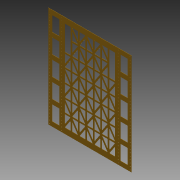
# Autodesk Inventor part: Cover Nick
Saved by Autodesk Inventor 2014 SP1 (Build 180222100, 222)
## iProperties
Created: 2014-01-21
Part Number: Cover Nick
Material: Aluminum 6061
Document SubType Name: Sheet Metal
Designer: Nick
Density: 2.71 g/cm^3
Sheet Metal Rule: Default
Appearance: Brass - Satin
Mass: 2078.93 g
Surface Area: 7373.94 cm^2
Volume: 767.135 cm^3
Author: Nick
Autodesk Inventor part; units mm, degrees
(part 1 of 2)
ref_plane "YZ Plane" through (0, 0, 0) normal (1, 0, 0) x (0, 1, 0)
ref_plane "XZ Plane" through (0, 0, 0) normal (0, 1, 0) x (-1, 0, 0)
ref_plane "XY Plane" through (0, 0, 0) normal (0, 0, 1) x (1, 0, 0)
sketch "Sketch1" plane through (0, 0, 0) normal (0, 0, 1) x (1, 0, 0)
  line L0 (0, 0) -> (711.2, 0)
  line L1 (711.2, 0) -> (711.2, -863.6)
  line L2 (711.2, -863.6) -> (0, -863.6)
  line L3 (0, -863.6) -> (0, 0)
  line L4 (139.7, -50.0761) -> (139.7, -112.6148)
  line L5 (145.5168, -114.376) -> (187.2092, -51.8373)
  line L6 (184.5675, -46.9011) -> (142.875, -46.9011)
  line L7 (190.5, -69.7865) -> (190.5, -142.8115)
  line L8 (187.325, -145.9865) -> (145.6325, -145.9865)
  line L9 (142.9908, -141.0503) -> (190.5, -69.7865)
  line L10 (196.85, 58.9554) -> (196.85, -325.5512) construction
  line L11 (254, -50.0761) -> (254, -112.6148)
  line L12 (248.1832, -114.376) -> (206.4908, -51.8373)
  line L13 (209.1325, -46.9011) -> (250.825, -46.9011)
  line L14 (203.2, -80.2728) -> (203.2, -142.8115)
  line L15 (206.375, -145.9865) -> (248.0675, -145.9865)
  line L16 (250.7092, -141.0503) -> (209.0168, -78.5116)
  arc A0 (142.875, -46.9011) -> (139.7, -50.0761) centre (142.875, -50.0761) ccw
  arc A1 (139.7, -112.6148) -> (145.5168, -114.376) centre (142.875, -112.6148) ccw
  arc A2 (187.2092, -51.8373) -> (184.5675, -46.9011) centre (184.5675, -50.0761) ccw
  arc A3 (209.1325, -46.9011) -> (206.4908, -51.8373) centre (209.1325, -50.0761) ccw
  arc A4 (254, -50.0761) -> (250.825, -46.9011) centre (250.825, -50.0761) ccw
  arc A5 (248.1832, -114.376) -> (254, -112.6148) centre (250.825, -112.6148) ccw
  arc A6 (248.0675, -145.9865) -> (250.7092, -141.0503) centre (248.0675, -142.8115) ccw
  arc A7 (209.0168, -78.5116) -> (203.2, -80.2728) centre (206.375, -80.2728) ccw
  arc A8 (203.2, -142.8115) -> (206.375, -145.9865) centre (206.375, -142.8115) ccw
  arc A9 (187.325, -145.9865) -> (190.5, -142.8115) centre (187.325, -142.8115) ccw
  arc A10 (142.9908, -141.0503) -> (145.6325, -145.9865) centre (145.6325, -142.8115) ccw
  line L17 (88.986, -152.3365) -> (322.9088, -152.3365) construction
  line L18 (139.7, -254.5969) -> (139.7, -192.0582)
  line L19 (145.5168, -190.297) -> (187.2092, -252.8357)
  line L20 (184.5675, -257.7719) -> (142.875, -257.7719)
  line L21 (190.5, -234.8865) -> (190.5, -161.8615)
  line L22 (187.325, -158.6865) -> (145.6325, -158.6865)
  line L23 (142.9908, -163.6227) -> (190.5, -234.8865)
  line L24 (209.1325, -257.7719) -> (250.825, -257.7719)
  line L25 (254, -254.5969) -> (254, -192.0582)
  line L26 (248.1832, -190.297) -> (206.4908, -252.8357)
  line L27 (206.375, -158.6865) -> (248.0675, -158.6865)
  line L28 (250.7092, -163.6227) -> (209.0168, -226.1614)
  line L29 (203.2, -224.4002) -> (203.2, -161.8615)
  arc A11 (139.7, -254.5969) -> (142.875, -257.7719) centre (142.875, -254.5969) ccw
  arc A12 (145.5168, -190.297) -> (139.7, -192.0582) centre (142.875, -192.0582) ccw
  arc A13 (184.5675, -257.7719) -> (187.2092, -252.8357) centre (184.5675, -254.5969) ccw
  arc A14 (206.4908, -252.8357) -> (209.1325, -257.7719) centre (209.1325, -254.5969) ccw
  arc A15 (250.825, -257.7719) -> (254, -254.5969) centre (250.825, -254.5969) ccw
  arc A16 (254, -192.0582) -> (248.1832, -190.297) centre (250.825, -192.0582) ccw
  arc A17 (250.7092, -163.6227) -> (248.0675, -158.6865) centre (248.0675, -161.8615) ccw
  arc A18 (203.2, -224.4002) -> (209.0168, -226.1614) centre (206.375, -224.4002) ccw
  arc A19 (206.375, -158.6865) -> (203.2, -161.8615) centre (206.375, -161.8615) ccw
  arc A20 (190.5, -161.8615) -> (187.325, -158.6865) centre (187.325, -161.8615) ccw
  arc A21 (145.6325, -158.6865) -> (142.9908, -163.6227) centre (145.6325, -161.8615) ccw
  line L30 (266.7, -50.0761) -> (266.7, -112.6148)
  line L31 (272.5168, -114.376) -> (314.2092, -51.8373)
  line L32 (311.5675, -46.9011) -> (269.875, -46.9011)
  line L33 (317.5, -69.7865) -> (317.5, -142.8115)
  line L34 (314.325, -145.9865) -> (272.6325, -145.9865)
  line L35 (269.9908, -141.0503) -> (317.5, -69.7865)
  line L36 (336.1325, -46.9011) -> (377.825, -46.9011)
  line L37 (381, -50.0761) -> (381, -112.6148)
  line L38 (375.1832, -114.376) -> (333.4908, -51.8373)
  line L39 (333.375, -145.9865) -> (375.0675, -145.9865)
  line L40 (377.7092, -141.0503) -> (336.0168, -78.5116)
  line L41 (330.2, -80.2728) -> (330.2, -142.8115)
  arc A22 (269.875, -46.9011) -> (266.7, -50.0761) centre (269.875, -50.0761) ccw
  arc A23 (266.7, -112.6148) -> (272.5168, -114.376) centre (269.875, -112.6148) ccw
  arc A24 (314.2092, -51.8373) -> (311.5675, -46.9011) centre (311.5675, -50.0761) ccw
  arc A25 (336.1325, -46.9011) -> (333.4908, -51.8373) centre (336.1325, -50.0761) ccw
  arc A26 (381, -50.0761) -> (377.825, -46.9011) centre (377.825, -50.0761) ccw
  arc A27 (375.1832, -114.376) -> (381, -112.6148) centre (377.825, -112.6148) ccw
  arc A28 (375.0675, -145.9865) -> (377.7092, -141.0503) centre (375.0675, -142.8115) ccw
  arc A29 (336.0168, -78.5116) -> (330.2, -80.2728) centre (333.375, -80.2728) ccw
  arc A30 (330.2, -142.8115) -> (333.375, -145.9865) centre (333.375, -142.8115) ccw
  arc A31 (314.325, -145.9865) -> (317.5, -142.8115) centre (314.325, -142.8115) ccw
  arc A32 (269.9908, -141.0503) -> (272.6325, -145.9865) centre (272.6325, -142.8115) ccw
  line L42 (317.5, -234.8865) -> (317.5, -161.8615)
  line L43 (269.9908, -163.6227) -> (317.5, -234.8865)
  line L44 (272.5168, -190.297) -> (314.2092, -252.8357)
  line L45 (311.5675, -257.7719) -> (269.875, -257.7719)
  line L46 (266.7, -254.5969) -> (266.7, -192.0582)
  line L47 (330.2, -224.4002) -> (330.2, -161.8615)
  line L48 (314.325, -158.6865) -> (272.6325, -158.6865)
  arc A33 (317.5, -161.8615) -> (314.325, -158.6865) centre (314.325, -161.8615) ccw
  arc A34 (272.5168, -190.297) -> (266.7, -192.0582) centre (269.875, -192.0582) ccw
  arc A35 (272.6325, -158.6865) -> (269.9908, -163.6227) centre (272.6325, -161.8615) ccw
  arc A36 (330.2, -224.4002) -> (336.0168, -226.1614) centre (333.375, -224.4002) ccw
  arc A37 (333.375, -158.6865) -> (330.2, -161.8615) centre (333.375, -161.8615) ccw
  line L49 (375.1832, -190.297) -> (333.4908, -252.8357)
  line L50 (381, -254.5969) -> (381, -192.0582)
  line L51 (377.7092, -163.6227) -> (336.0168, -226.1614)
  line L52 (333.375, -158.6865) -> (375.0675, -158.6865)
  arc A38 (381, -192.0582) -> (375.1832, -190.297) centre (377.825, -192.0582) ccw
  arc A39 (377.7092, -163.6227) -> (375.0675, -158.6865) centre (375.0675, -161.8615) ccw
  arc A40 (266.7, -254.5969) -> (269.875, -257.7719) centre (269.875, -254.5969) ccw
  line L53 (336.1325, -257.7719) -> (377.825, -257.7719)
  arc A41 (311.5675, -257.7719) -> (314.2092, -252.8357) centre (311.5675, -254.5969) ccw
  arc A42 (377.825, -257.7719) -> (381, -254.5969) centre (377.825, -254.5969) ccw
  arc A43 (333.4908, -252.8357) -> (336.1325, -257.7719) centre (336.1325, -254.5969) ccw
  line L54 (393.7, -50.0761) -> (393.7, -112.6148)
  line L55 (399.5168, -114.376) -> (441.2092, -51.8373)
  line L56 (438.5675, -46.9011) -> (396.875, -46.9011)
  line L57 (444.5, -69.7865) -> (444.5, -142.8115)
  line L58 (441.325, -145.9865) -> (399.6325, -145.9865)
  line L59 (396.9908, -141.0503) -> (444.5, -69.7865)
  line L60 (463.1325, -46.9011) -> (504.825, -46.9011)
  line L61 (508, -50.0761) -> (508, -112.6148)
  line L62 (502.1832, -114.376) -> (460.4908, -51.8373)
  line L63 (460.375, -145.9865) -> (502.0675, -145.9865)
  line L64 (504.7092, -141.0503) -> (463.0168, -78.5116)
  line L65 (457.2, -80.2728) -> (457.2, -142.8115)
  arc A44 (396.875, -46.9011) -> (393.7, -50.0761) centre (396.875, -50.0761) ccw
  arc A45 (393.7, -112.6148) -> (399.5168, -114.376) centre (396.875, -112.6148) ccw
  arc A46 (441.2092, -51.8373) -> (438.5675, -46.9011) centre (438.5675, -50.0761) ccw
  arc A47 (463.1325, -46.9011) -> (460.4908, -51.8373) centre (463.1325, -50.0761) ccw
  arc A48 (508, -50.0761) -> (504.825, -46.9011) centre (504.825, -50.0761) ccw
  arc A49 (502.1832, -114.376) -> (508, -112.6148) centre (504.825, -112.6148) ccw
  arc A50 (502.0675, -145.9865) -> (504.7092, -141.0503) centre (502.0675, -142.8115) ccw
  arc A51 (463.0168, -78.5116) -> (457.2, -80.2728) centre (460.375, -80.2728) ccw
  arc A52 (457.2, -142.8115) -> (460.375, -145.9865) centre (460.375, -142.8115) ccw
  arc A53 (441.325, -145.9865) -> (444.5, -142.8115) centre (441.325, -142.8115) ccw
  arc A54 (396.9908, -141.0503) -> (399.6325, -145.9865) centre (399.6325, -142.8115) ccw
  line L66 (444.5, -234.8865) -> (444.5, -161.8615)
  line L67 (396.9908, -163.6227) -> (444.5, -234.8865)
  line L68 (399.5168, -190.297) -> (441.2092, -252.8357)
  line L69 (438.5675, -257.7719) -> (396.875, -257.7719)
  line L70 (393.7, -254.5969) -> (393.7, -192.0582)
  line L71 (457.2, -224.4002) -> (457.2, -161.8615)
  line L72 (441.325, -158.6865) -> (399.6325, -158.6865)
  arc A55 (444.5, -161.8615) -> (441.325, -158.6865) centre (441.325, -161.8615) ccw
  arc A56 (399.5168, -190.297) -> (393.7, -192.0582) centre (396.875, -192.0582) ccw
  arc A57 (399.6325, -158.6865) -> (396.9908, -163.6227) centre (399.6325, -161.8615) ccw
  arc A58 (457.2, -224.4002) -> (463.0168, -226.1614) centre (460.375, -224.4002) ccw
  arc A59 (460.375, -158.6865) -> (457.2, -161.8615) centre (460.375, -161.8615) ccw
  line L73 (502.1832, -190.297) -> (460.4908, -252.8357)
  line L74 (508, -254.5969) -> (508, -192.0582)
  line L75 (504.7092, -163.6227) -> (463.0168, -226.1614)
  line L76 (460.375, -158.6865) -> (502.0675, -158.6865)
  arc A60 (508, -192.0582) -> (502.1832, -190.297) centre (504.825, -192.0582) ccw
  arc A61 (504.7092, -163.6227) -> (502.0675, -158.6865) centre (502.0675, -161.8615) ccw
  arc A62 (393.7, -254.5969) -> (396.875, -257.7719) centre (396.875, -254.5969) ccw
  line L77 (463.1325, -257.7719) -> (504.825, -257.7719)
  arc A63 (438.5675, -257.7719) -> (441.2092, -252.8357) centre (438.5675, -254.5969) ccw
  arc A64 (504.825, -257.7719) -> (508, -254.5969) centre (504.825, -254.5969) ccw
  arc A65 (460.4908, -252.8357) -> (463.1325, -257.7719) centre (463.1325, -254.5969) ccw
  line L78 (139.7, -273.6469) -> (139.7, -336.1856)
  line L79 (145.5168, -337.9468) -> (187.2092, -275.4081)
  line L80 (184.5675, -270.4719) -> (142.875, -270.4719)
  line L81 (190.5, -293.3573) -> (190.5, -366.3823)
  line L82 (187.325, -369.5573) -> (145.6325, -369.5573)
  line L83 (142.9908, -364.6211) -> (190.5, -293.3573)
  line L84 (209.1325, -270.4719) -> (250.825, -270.4719)
  line L85 (254, -273.6469) -> (254, -336.1856)
  line L86 (248.1832, -337.9468) -> (206.4908, -275.4081)
  line L87 (206.375, -369.5573) -> (248.0675, -369.5573)
  line L88 (250.7092, -364.6211) -> (209.0168, -302.0824)
  line L89 (203.2, -303.8436) -> (203.2, -366.3823)
  arc A66 (142.875, -270.4719) -> (139.7, -273.6469) centre (142.875, -273.6469) ccw
  arc A67 (139.7, -336.1856) -> (145.5168, -337.9468) centre (142.875, -336.1856) ccw
  arc A68 (187.2092, -275.4081) -> (184.5675, -270.4719) centre (184.5675, -273.6469) ccw
  arc A69 (209.1325, -270.4719) -> (206.4908, -275.4081) centre (209.1325, -273.6469) ccw
  arc A70 (254, -273.6469) -> (250.825, -270.4719) centre (250.825, -273.6469) ccw
  arc A71 (248.1832, -337.9468) -> (254, -336.1856) centre (250.825, -336.1856) ccw
  arc A72 (248.0675, -369.5573) -> (250.7092, -364.6211) centre (248.0675, -366.3823) ccw
  arc A73 (209.0168, -302.0824) -> (203.2, -303.8436) centre (206.375, -303.8436) ccw
  arc A74 (203.2, -366.3823) -> (206.375, -369.5573) centre (206.375, -366.3823) ccw
  arc A75 (187.325, -369.5573) -> (190.5, -366.3823) centre (187.325, -366.3823) ccw
  arc A76 (142.9908, -364.6211) -> (145.6325, -369.5573) centre (145.6325, -366.3823) ccw
  line L90 (190.5, -458.4573) -> (190.5, -385.4323)
  line L91 (142.9908, -387.1935) -> (190.5, -458.4573)
  line L92 (145.5168, -413.8678) -> (187.2092, -476.4065)
  line L93 (184.5675, -481.3427) -> (142.875, -481.3427)
  line L94 (139.7, -478.1677) -> (139.7, -415.629)
  line L95 (203.2, -447.971) -> (203.2, -385.4323)
  line L96 (187.325, -382.2573) -> (145.6325, -382.2573)
  arc A77 (190.5, -385.4323) -> (187.325, -382.2573) centre (187.325, -385.4323) ccw
  arc A78 (145.5168, -413.8678) -> (139.7, -415.629) centre (142.875, -415.629) ccw
  arc A79 (145.6325, -382.2573) -> (142.9908, -387.1935) centre (145.6325, -385.4323) ccw
  arc A80 (203.2, -447.971) -> (209.0168, -449.7322) centre (206.375, -447.971) ccw
  arc A81 (206.375, -382.2573) -> (203.2, -385.4323) centre (206.375, -385.4323) ccw
  line L97 (248.1832, -413.8678) -> (206.4908, -476.4065)
  line L98 (254, -478.1677) -> (254, -415.629)
  line L99 (250.7092, -387.1935) -> (209.0168, -449.7322)
  line L100 (206.375, -382.2573) -> (248.0675, -382.2573)
  arc A82 (254, -415.629) -> (248.1832, -413.8678) centre (250.825, -415.629) ccw
  arc A83 (250.7092, -387.1935) -> (248.0675, -382.2573) centre (248.0675, -385.4323) ccw
  arc A84 (139.7, -478.1677) -> (142.875, -481.3427) centre (142.875, -478.1677) ccw
  line L101 (209.1325, -481.3427) -> (250.825, -481.3427)
  arc A85 (184.5675, -481.3427) -> (187.2092, -476.4065) centre (184.5675, -478.1677) ccw
  arc A86 (250.825, -481.3427) -> (254, -478.1677) centre (250.825, -478.1677) ccw
  arc A87 (206.4908, -476.4065) -> (209.1325, -481.3427) centre (209.1325, -478.1677) ccw
  line L102 (266.7, -273.6469) -> (266.7, -336.1856)
  line L103 (272.5168, -337.9468) -> (314.2092, -275.4081)
  line L104 (311.5675, -270.4719) -> (269.875, -270.4719)
  line L105 (317.5, -293.3573) -> (317.5, -366.3823)
  line L106 (314.325, -369.5573) -> (272.6325, -369.5573)
  line L107 (269.9908, -364.6211) -> (317.5, -293.3573)
  line L108 (336.1325, -270.4719) -> (377.825, -270.4719)
  line L109 (381, -273.6469) -> (381, -336.1856)
  line L110 (375.1832, -337.9468) -> (333.4908, -275.4081)
  line L111 (333.375, -369.5573) -> (375.0675, -369.5573)
  line L112 (377.7092, -364.6211) -> (336.0168, -302.0824)
  line L113 (330.2, -303.8436) -> (330.2, -366.3823)
  arc A88 (269.875, -270.4719) -> (266.7, -273.6469) centre (269.875, -273.6469) ccw
  arc A89 (266.7, -336.1856) -> (272.5168, -337.9468) centre (269.875, -336.1856) ccw
  arc A90 (314.2092, -275.4081) -> (311.5675, -270.4719) centre (311.5675, -273.6469) ccw
  arc A91 (336.1325, -270.4719) -> (333.4908, -275.4081) centre (336.1325, -273.6469) ccw
  arc A92 (381, -273.6469) -> (377.825, -270.4719) centre (377.825, -273.6469) ccw
  arc A93 (375.1832, -337.9468) -> (381, -336.1856) centre (377.825, -336.1856) ccw
  arc A94 (375.0675, -369.5573) -> (377.7092, -364.6211) centre (375.0675, -366.3823) ccw
  arc A95 (336.0168, -302.0824) -> (330.2, -303.8436) centre (333.375, -303.8436) ccw
  arc A96 (330.2, -366.3823) -> (333.375, -369.5573) centre (333.375, -366.3823) ccw
  arc A97 (314.325, -369.5573) -> (317.5, -366.3823) centre (314.325, -366.3823) ccw
  arc A98 (269.9908, -364.6211) -> (272.6325, -369.5573) centre (272.6325, -366.3823) ccw
  line L114 (317.5, -458.4573) -> (317.5, -385.4323)
  line L115 (269.9908, -387.1935) -> (317.5, -458.4573)
  line L116 (272.5168, -413.8678) -> (314.2092, -476.4065)
  line L117 (311.5675, -481.3427) -> (269.875, -481.3427)
  line L118 (266.7, -478.1677) -> (266.7, -415.629)
  line L119 (330.2, -447.971) -> (330.2, -385.4323)
  line L120 (314.325, -382.2573) -> (272.6325, -382.2573)
  arc A99 (317.5, -385.4323) -> (314.325, -382.2573) centre (314.325, -385.4323) ccw
  arc A100 (272.5168, -413.8678) -> (266.7, -415.629) centre (269.875, -415.629) ccw
  arc A101 (272.6325, -382.2573) -> (269.9908, -387.1935) centre (272.6325, -385.4323) ccw
  arc A102 (330.2, -447.971) -> (336.0168, -449.7322) centre (333.375, -447.971) ccw
  arc A103 (333.375, -382.2573) -> (330.2, -385.4323) centre (333.375, -385.4323) ccw
  line L121 (375.1832, -413.8678) -> (333.4908, -476.4065)
  line L122 (381, -478.1677) -> (381, -415.629)
  line L123 (377.7092, -387.1935) -> (336.0168, -449.7322)
  line L124 (333.375, -382.2573) -> (375.0675, -382.2573)
  arc A104 (381, -415.629) -> (375.1832, -413.8678) centre (377.825, -415.629) ccw
  arc A105 (377.7092, -387.1935) -> (375.0675, -382.2573) centre (375.0675, -385.4323) ccw
  arc A106 (266.7, -478.1677) -> (269.875, -481.3427) centre (269.875, -478.1677) ccw
  line L125 (336.1325, -481.3427) -> (377.825, -481.3427)
  arc A107 (311.5675, -481.3427) -> (314.2092, -476.4065) centre (311.5675, -478.1677) ccw
  arc A108 (377.825, -481.3427) -> (381, -478.1677) centre (377.825, -478.1677) ccw
  arc A109 (333.4908, -476.4065) -> (336.1325, -481.3427) centre (336.1325, -478.1677) ccw
  line L126 (393.7, -273.6469) -> (393.7, -336.1856)
  line L127 (399.5168, -337.9468) -> (441.2092, -275.4081)
  line L128 (438.5675, -270.4719) -> (396.875, -270.4719)
  line L129 (444.5, -293.3573) -> (444.5, -366.3823)
  line L130 (441.325, -369.5573) -> (399.6325, -369.5573)
  line L131 (396.9908, -364.6211) -> (444.5, -293.3573)
  line L132 (463.1325, -270.4719) -> (504.825, -270.4719)
  line L133 (508, -273.6469) -> (508, -336.1856)
  line L134 (502.1832, -337.9468) -> (460.4908, -275.4081)
  line L135 (460.375, -369.5573) -> (502.0675, -369.5573)
  line L136 (504.7092, -364.6211) -> (463.0168, -302.0824)
  line L137 (457.2, -303.8436) -> (457.2, -366.3823)
  arc A110 (396.875, -270.4719) -> (393.7, -273.6469) centre (396.875, -273.6469) ccw
  arc A111 (393.7, -336.1856) -> (399.5168, -337.9468) centre (396.875, -336.1856) ccw
  arc A112 (441.2092, -275.4081) -> (438.5675, -270.4719) centre (438.5675, -273.6469) ccw
  arc A113 (463.1325, -270.4719) -> (460.4908, -275.4081) centre (463.1325, -273.6469) ccw
  arc A114 (508, -273.6469) -> (504.825, -270.4719) centre (504.825, -273.6469) ccw
  arc A115 (502.1832, -337.9468) -> (508, -336.1856) centre (504.825, -336.1856) ccw
  arc A116 (502.0675, -369.5573) -> (504.7092, -364.6211) centre (502.0675, -366.3823) ccw
  arc A117 (463.0168, -302.0824) -> (457.2, -303.8436) centre (460.375, -303.8436) ccw
  arc A118 (457.2, -366.3823) -> (460.375, -369.5573) centre (460.375, -366.3823) ccw
  arc A119 (441.325, -369.5573) -> (444.5, -366.3823) centre (441.325, -366.3823) ccw
  arc A120 (396.9908, -364.6211) -> (399.6325, -369.5573) centre (399.6325, -366.3823) ccw
  line L138 (444.5, -458.4573) -> (444.5, -385.4323)
  line L139 (396.9908, -387.1935) -> (444.5, -458.4573)
  line L140 (399.5168, -413.8678) -> (441.2092, -476.4065)
  line L141 (438.5675, -481.3427) -> (396.875, -481.3427)
  line L142 (393.7, -478.1677) -> (393.7, -415.629)
  line L143 (457.2, -447.971) -> (457.2, -385.4323)
  line L144 (441.325, -382.2573) -> (399.6325, -382.2573)
  arc A121 (444.5, -385.4323) -> (441.325, -382.2573) centre (441.325, -385.4323) ccw
  arc A122 (399.5168, -413.8678) -> (393.7, -415.629) centre (396.875, -415.629) ccw
  arc A123 (399.6325, -382.2573) -> (396.9908, -387.1935) centre (399.6325, -385.4323) ccw
  arc A124 (457.2, -447.971) -> (463.0168, -449.7322) centre (460.375, -447.971) ccw
  arc A125 (460.375, -382.2573) -> (457.2, -385.4323) centre (460.375, -385.4323) ccw
  line L145 (502.1832, -413.8678) -> (460.4908, -476.4065)
  line L146 (508, -478.1677) -> (508, -415.629)
  line L147 (504.7092, -387.1935) -> (463.0168, -449.7322)
  line L148 (460.375, -382.2573) -> (502.0675, -382.2573)
  arc A126 (508, -415.629) -> (502.1832, -413.8678) centre (504.825, -415.629) ccw
  arc A127 (504.7092, -387.1935) -> (502.0675, -382.2573) centre (502.0675, -385.4323) ccw
  arc A128 (393.7, -478.1677) -> (396.875, -481.3427) centre (396.875, -478.1677) ccw
  line L149 (463.1325, -481.3427) -> (504.825, -481.3427)
  arc A129 (438.5675, -481.3427) -> (441.2092, -476.4065) centre (438.5675, -478.1677) ccw
  arc A130 (504.825, -481.3427) -> (508, -478.1677) centre (504.825, -478.1677) ccw
  arc A131 (460.4908, -476.4065) -> (463.1325, -481.3427) centre (463.1325, -478.1677) ccw
  line L150 (139.7, -497.2177) -> (139.7, -559.7564)
  line L151 (145.5168, -561.5176) -> (187.2092, -498.9789)
  line L152 (184.5675, -494.0427) -> (142.875, -494.0427)
  line L153 (190.5, -516.9281) -> (190.5, -589.9531)
  line L154 (187.325, -593.1281) -> (145.6325, -593.1281)
  line L155 (142.9908, -588.1919) -> (190.5, -516.9281)
  line L156 (209.1325, -494.0427) -> (250.825, -494.0427)
  line L157 (254, -497.2177) -> (254, -559.7564)
  line L158 (248.1832, -561.5176) -> (206.4908, -498.9789)
  line L159 (206.375, -593.1281) -> (248.0675, -593.1281)
  line L160 (250.7092, -588.1919) -> (209.0168, -525.6532)
  line L161 (203.2, -527.4144) -> (203.2, -589.9531)
  arc A132 (142.875, -494.0427) -> (139.7, -497.2177) centre (142.875, -497.2177) ccw
  arc A133 (139.7, -559.7564) -> (145.5168, -561.5176) centre (142.875, -559.7564) ccw
  arc A134 (187.2092, -498.9789) -> (184.5675, -494.0427) centre (184.5675, -497.2177) ccw
  arc A135 (209.1325, -494.0427) -> (206.4908, -498.9789) centre (209.1325, -497.2177) ccw
  arc A136 (254, -497.2177) -> (250.825, -494.0427) centre (250.825, -497.2177) ccw
  arc A137 (248.1832, -561.5176) -> (254, -559.7564) centre (250.825, -559.7564) ccw
  arc A138 (248.0675, -593.1281) -> (250.7092, -588.1919) centre (248.0675, -589.9531) ccw
  arc A139 (209.0168, -525.6532) -> (203.2, -527.4144) centre (206.375, -527.4144) ccw
  arc A140 (203.2, -589.9531) -> (206.375, -593.1281) centre (206.375, -589.9531) ccw
  arc A141 (187.325, -593.1281) -> (190.5, -589.9531) centre (187.325, -589.9531) ccw
  arc A142 (142.9908, -588.1919) -> (145.6325, -593.1281) centre (145.6325, -589.9531) ccw
  line L162 (190.5, -682.0281) -> (190.5, -609.0031)
  line L163 (142.9908, -610.7643) -> (190.5, -682.0281)
  line L164 (145.5168, -637.4386) -> (187.2092, -699.9773)
  line L165 (184.5675, -704.9135) -> (142.875, -704.9135)
  line L166 (139.7, -701.7385) -> (139.7, -639.1998)
  line L167 (203.2, -671.5418) -> (203.2, -609.0031)
  line L168 (187.325, -605.8281) -> (145.6325, -605.8281)
  arc A143 (190.5, -609.0031) -> (187.325, -605.8281) centre (187.325, -609.0031) ccw
  arc A144 (145.5168, -637.4386) -> (139.7, -639.1998) centre (142.875, -639.1998) ccw
  arc A145 (145.6325, -605.8281) -> (142.9908, -610.7643) centre (145.6325, -609.0031) ccw
  arc A146 (203.2, -671.5418) -> (209.0168, -673.303) centre (206.375, -671.5418) ccw
  arc A147 (206.375, -605.8281) -> (203.2, -609.0031) centre (206.375, -609.0031) ccw
  line L169 (248.1832, -637.4386) -> (206.4908, -699.9773)
  line L170 (254, -701.7385) -> (254, -639.1998)
  line L171 (250.7092, -610.7643) -> (209.0168, -673.303)
  line L172 (206.375, -605.8281) -> (248.0675, -605.8281)
  arc A148 (254, -639.1998) -> (248.1832, -637.4386) centre (250.825, -639.1998) ccw
  arc A149 (250.7092, -610.7643) -> (248.0675, -605.8281) centre (248.0675, -609.0031) ccw
  arc A150 (139.7, -701.7385) -> (142.875, -704.9135) centre (142.875, -701.7385) ccw
  line L173 (209.1325, -704.9135) -> (250.825, -704.9135)
  arc A151 (184.5675, -704.9135) -> (187.2092, -699.9773) centre (184.5675, -701.7385) ccw
  arc A152 (250.825, -704.9135) -> (254, -701.7385) centre (250.825, -701.7385) ccw
  arc A153 (206.4908, -699.9773) -> (209.1325, -704.9135) centre (209.1325, -701.7385) ccw
  line L174 (266.7, -497.2177) -> (266.7, -559.7564)
  line L175 (272.5168, -561.5176) -> (314.2092, -498.9789)
  line L176 (311.5675, -494.0427) -> (269.875, -494.0427)
  line L177 (317.5, -516.9281) -> (317.5, -589.9531)
  line L178 (314.325, -593.1281) -> (272.6325, -593.1281)
  line L179 (269.9908, -588.1919) -> (317.5, -516.9281)
  line L180 (336.1325, -494.0427) -> (377.825, -494.0427)
  line L181 (381, -497.2177) -> (381, -559.7564)
  line L182 (375.1832, -561.5176) -> (333.4908, -498.9789)
  line L183 (333.375, -593.1281) -> (375.0675, -593.1281)
  line L184 (377.7092, -588.1919) -> (336.0168, -525.6532)
  line L185 (330.2, -527.4144) -> (330.2, -589.9531)
  arc A154 (269.875, -494.0427) -> (266.7, -497.2177) centre (269.875, -497.2177) ccw
  arc A155 (266.7, -559.7564) -> (272.5168, -561.5176) centre (269.875, -559.7564) ccw
  arc A156 (314.2092, -498.9789) -> (311.5675, -494.0427) centre (311.5675, -497.2177) ccw
  arc A157 (336.1325, -494.0427) -> (333.4908, -498.9789) centre (336.1325, -497.2177) ccw
  arc A158 (381, -497.2177) -> (377.825, -494.0427) centre (377.825, -497.2177) ccw
  arc A159 (375.1832, -561.5176) -> (381, -559.7564) centre (377.825, -559.7564) ccw
  arc A160 (375.0675, -593.1281) -> (377.7092, -588.1919) centre (375.0675, -589.9531) ccw
  arc A161 (336.0168, -525.6532) -> (330.2, -527.4144) centre (333.375, -527.4144) ccw
  arc A162 (330.2, -589.9531) -> (333.375, -593.1281) centre (333.375, -589.9531) ccw
  arc A163 (314.325, -593.1281) -> (317.5, -589.9531) centre (314.325, -589.9531) ccw
  arc A164 (269.9908, -588.1919) -> (272.6325, -593.1281) centre (272.6325, -589.9531) ccw
  line L186 (317.5, -682.0281) -> (317.5, -609.0031)
  line L187 (269.9908, -610.7643) -> (317.5, -682.0281)
  line L188 (272.5168, -637.4386) -> (314.2092, -699.9773)
  line L189 (311.5675, -704.9135) -> (269.875, -704.9135)
  line L190 (266.7, -701.7385) -> (266.7, -639.1998)
  line L191 (330.2, -671.5418) -> (330.2, -609.0031)
  line L192 (314.325, -605.8281) -> (272.6325, -605.8281)
  arc A165 (317.5, -609.0031) -> (314.325, -605.8281) centre (314.325, -609.0031) ccw
  arc A166 (272.5168, -637.4386) -> (266.7, -639.1998) centre (269.875, -639.1998) ccw
  arc A167 (272.6325, -605.8281) -> (269.9908, -610.7643) centre (272.6325, -609.0031) ccw
  arc A168 (330.2, -671.5418) -> (336.0168, -673.303) centre (333.375, -671.5418) ccw
  arc A169 (333.375, -605.8281) -> (330.2, -609.0031) centre (333.375, -609.0031) ccw
  line L193 (375.1832, -637.4386) -> (333.4908, -699.9773)
  line L194 (381, -701.7385) -> (381, -639.1998)
  line L195 (377.7092, -610.7643) -> (336.0168, -673.303)
  line L196 (333.375, -605.8281) -> (375.0675, -605.8281)
  arc A170 (381, -639.1998) -> (375.1832, -637.4386) centre (377.825, -639.1998) ccw
  arc A171 (377.7092, -610.7643) -> (375.0675, -605.8281) centre (375.0675, -609.0031) ccw
  arc A172 (266.7, -701.7385) -> (269.875, -704.9135) centre (269.875, -701.7385) ccw
  line L197 (336.1325, -704.9135) -> (377.825, -704.9135)
  arc A173 (311.5675, -704.9135) -> (314.2092, -699.9773) centre (311.5675, -701.7385) ccw
  arc A174 (377.825, -704.9135) -> (381, -701.7385) centre (377.825, -701.7385) ccw
  arc A175 (333.4908, -699.9773) -> (336.1325, -704.9135) centre (336.1325, -701.7385) ccw
  line L198 (393.7, -497.2177) -> (393.7, -559.7564)
  line L199 (399.5168, -561.5176) -> (441.2092, -498.9789)
  line L200 (438.5675, -494.0427) -> (396.875, -494.0427)
  line L201 (444.5, -516.9281) -> (444.5, -589.9531)
  line L202 (441.325, -593.1281) -> (399.6325, -593.1281)
  line L203 (396.9908, -588.1919) -> (444.5, -516.9281)
  line L204 (463.1325, -494.0427) -> (504.825, -494.0427)
  line L205 (508, -497.2177) -> (508, -559.7564)
  line L206 (502.1832, -561.5176) -> (460.4908, -498.9789)
  line L207 (460.375, -593.1281) -> (502.0675, -593.1281)
  line L208 (504.7092, -588.1919) -> (463.0168, -525.6532)
  line L209 (457.2, -527.4144) -> (457.2, -589.9531)
  arc A176 (396.875, -494.0427) -> (393.7, -497.2177) centre (396.875, -497.2177) ccw
  arc A177 (393.7, -559.7564) -> (399.5168, -561.5176) centre (396.875, -559.7564) ccw
  arc A178 (441.2092, -498.9789) -> (438.5675, -494.0427) centre (438.5675, -497.2177) ccw
  arc A179 (463.1325, -494.0427) -> (460.4908, -498.9789) centre (463.1325, -497.2177) ccw
  arc A180 (508, -497.2177) -> (504.825, -494.0427) centre (504.825, -497.2177) ccw
  arc A181 (502.1832, -561.5176) -> (508, -559.7564) centre (504.825, -559.7564) ccw
  arc A182 (502.0675, -593.1281) -> (504.7092, -588.1919) centre (502.0675, -589.9531) ccw
  arc A183 (463.0168, -525.6532) -> (457.2, -527.4144) centre (460.375, -527.4144) ccw
  arc A184 (457.2, -589.9531) -> (460.375, -593.1281) centre (460.375, -589.9531) ccw
  arc A185 (441.325, -593.1281) -> (444.5, -589.9531) centre (441.325, -589.9531) ccw
  arc A186 (396.9908, -588.1919) -> (399.6325, -593.1281) centre (399.6325, -589.9531) ccw
  line L210 (444.5, -682.0281) -> (444.5, -609.0031)
  line L211 (396.9908, -610.7643) -> (444.5, -682.0281)
  line L212 (399.5168, -637.4386) -> (441.2092, -699.9773)
  line L213 (438.5675, -704.9135) -> (396.875, -704.9135)
  line L214 (393.7, -701.7385) -> (393.7, -639.1998)
  line L215 (457.2, -671.5418) -> (457.2, -609.0031)
  line L216 (441.325, -605.8281) -> (399.6325, -605.8281)
  arc A187 (444.5, -609.0031) -> (441.325, -605.8281) centre (441.325, -609.0031) ccw
  arc A188 (399.5168, -637.4386) -> (393.7, -639.1998) centre (396.875, -639.1998) ccw
  arc A189 (399.6325, -605.8281) -> (396.9908, -610.7643) centre (399.6325, -609.0031) ccw
  arc A190 (457.2, -671.5418) -> (463.0168, -673.303) centre (460.375, -671.5418) ccw
  arc A191 (460.375, -605.8281) -> (457.2, -609.0031) centre (460.375, -609.0031) ccw
  line L217 (502.1832, -637.4386) -> (460.4908, -699.9773)
  line L218 (508, -701.7385) -> (508, -639.1998)
  line L219 (504.7092, -610.7643) -> (463.0168, -673.303)
  line L220 (460.375, -605.8281) -> (502.0675, -605.8281)
  arc A192 (508, -639.1998) -> (502.1832, -637.4386) centre (504.825, -639.1998) ccw
  arc A193 (504.7092, -610.7643) -> (502.0675, -605.8281) centre (502.0675, -609.0031) ccw
  arc A194 (393.7, -701.7385) -> (396.875, -704.9135) centre (396.875, -701.7385) ccw
  line L221 (463.1325, -704.9135) -> (504.825, -704.9135)
  arc A195 (438.5675, -704.9135) -> (441.2092, -699.9773) centre (438.5675, -701.7385) ccw
  arc A196 (504.825, -704.9135) -> (508, -701.7385) centre (504.825, -701.7385) ccw
  arc A197 (460.4908, -699.9773) -> (463.1325, -704.9135) centre (463.1325, -701.7385) ccw
  line L222 (514.35, 75.032) -> (514.35, -808.2969) construction
  arc A198 (571.5, -80.2728) -> (565.6832, -78.5116) centre (568.325, -80.2728) ccw
  arc A199 (568.2092, -51.8373) -> (565.5675, -46.9011) centre (565.5675, -50.0761) ccw
  line L223 (565.5675, -46.9011) -> (523.875, -46.9011)
  arc A200 (523.875, -46.9011) -> (520.7, -50.0761) centre (523.875, -50.0761) ccw
  line L224 (526.5168, -114.376) -> (568.2092, -51.8373)
  arc A201 (520.7, -112.6148) -> (526.5168, -114.376) centre (523.875, -112.6148) ccw
  line L225 (520.7, -50.0761) -> (520.7, -112.6148)
  arc A202 (568.325, -145.9865) -> (571.5, -142.8115) centre (568.325, -142.8115) ccw
  line L226 (571.5, -80.2728) -> (571.5, -142.8115)
  line L227 (568.325, -145.9865) -> (526.6325, -145.9865)
  arc A203 (523.9908, -141.0503) -> (526.6325, -145.9865) centre (526.6325, -142.8115) ccw
  line L228 (523.9908, -141.0503) -> (565.6832, -78.5116)
  arc A204 (571.5, -161.8615) -> (568.325, -158.6865) centre (568.325, -161.8615) ccw
  line L229 (571.5, -224.4002) -> (571.5, -161.8615)
  arc A205 (565.6832, -226.1614) -> (571.5, -224.4002) centre (568.325, -224.4002) ccw
  line L230 (568.325, -158.6865) -> (526.6325, -158.6865)
  arc A206 (526.6325, -158.6865) -> (523.9908, -163.6227) centre (526.6325, -161.8615) ccw
  line L231 (523.9908, -163.6227) -> (565.6832, -226.1614)
  arc A207 (526.5168, -190.297) -> (520.7, -192.0582) centre (523.875, -192.0582) ccw
  line L232 (526.5168, -190.297) -> (568.2092, -252.8357)
  line L233 (520.7, -254.5969) -> (520.7, -192.0582)
  arc A208 (520.7, -254.5969) -> (523.875, -257.7719) centre (523.875, -254.5969) ccw
  line L234 (565.5675, -257.7719) -> (523.875, -257.7719)
  arc A209 (565.5675, -257.7719) -> (568.2092, -252.8357) centre (565.5675, -254.5969) ccw
  arc A210 (571.5, -303.8436) -> (565.6832, -302.0824) centre (568.325, -303.8436) ccw
  arc A211 (568.2092, -275.4081) -> (565.5675, -270.4719) centre (565.5675, -273.6469) ccw
  line L235 (565.5675, -270.4719) -> (523.875, -270.4719)
  arc A212 (523.875, -270.4719) -> (520.7, -273.6469) centre (523.875, -273.6469) ccw
  line L236 (526.5168, -337.9468) -> (568.2092, -275.4081)
  arc A213 (520.7, -336.1856) -> (526.5168, -337.9468) centre (523.875, -336.1856) ccw
  line L237 (520.7, -273.6469) -> (520.7, -336.1856)
  arc A214 (568.325, -369.5573) -> (571.5, -366.3823) centre (568.325, -366.3823) ccw
  line L238 (571.5, -303.8436) -> (571.5, -366.3823)
  line L239 (568.325, -369.5573) -> (526.6325, -369.5573)
  arc A215 (523.9908, -364.6211) -> (526.6325, -369.5573) centre (526.6325, -366.3823) ccw
  line L240 (523.9908, -364.6211) -> (565.6832, -302.0824)
  arc A216 (571.5, -385.4323) -> (568.325, -382.2573) centre (568.325, -385.4323) ccw
  line L241 (571.5, -447.971) -> (571.5, -385.4323)
  arc A217 (565.6832, -449.7322) -> (571.5, -447.971) centre (568.325, -447.971) ccw
  line L242 (568.325, -382.2573) -> (526.6325, -382.2573)
  arc A218 (526.6325, -382.2573) -> (523.9908, -387.1935) centre (526.6325, -385.4323) ccw
  line L243 (523.9908, -387.1935) -> (565.6832, -449.7322)
  arc A219 (526.5168, -413.8678) -> (520.7, -415.629) centre (523.875, -415.629) ccw
  line L244 (526.5168, -413.8678) -> (568.2092, -476.4065)
  line L245 (520.7, -478.1677) -> (520.7, -415.629)
  arc A220 (520.7, -478.1677) -> (523.875, -481.3427) centre (523.875, -478.1677) ccw
  line L246 (565.5675, -481.3427) -> (523.875, -481.3427)
  arc A221 (565.5675, -481.3427) -> (568.2092, -476.4065) centre (565.5675, -478.1677) ccw
  arc A222 (571.5, -527.4144) -> (565.6832, -525.6532) centre (568.325, -527.4144) ccw
  arc A223 (568.2092, -498.9789) -> (565.5675, -494.0427) centre (565.5675, -497.2177) ccw
  line L247 (565.5675, -494.0427) -> (523.875, -494.0427)
  arc A224 (523.875, -494.0427) -> (520.7, -497.2177) centre (523.875, -497.2177) ccw
  line L248 (526.5168, -561.5176) -> (568.2092, -498.9789)
  arc A225 (520.7, -559.7564) -> (526.5168, -561.5176) centre (523.875, -559.7564) ccw
  line L249 (520.7, -497.2177) -> (520.7, -559.7564)
  arc A226 (568.325, -593.1281) -> (571.5, -589.9531) centre (568.325, -589.9531) ccw
  line L250 (571.5, -527.4144) -> (571.5, -589.9531)
  line L251 (568.325, -593.1281) -> (526.6325, -593.1281)
  arc A227 (523.9908, -588.1919) -> (526.6325, -593.1281) centre (526.6325, -589.9531) ccw
  line L252 (523.9908, -588.1919) -> (565.6832, -525.6532)
  arc A228 (571.5, -609.0031) -> (568.325, -605.8281) centre (568.325, -609.0031) ccw
  line L253 (571.5, -671.5418) -> (571.5, -609.0031)
  arc A229 (565.6832, -673.303) -> (571.5, -671.5418) centre (568.325, -671.5418) ccw
  line L254 (568.325, -605.8281) -> (526.6325, -605.8281)
  arc A230 (526.6325, -605.8281) -> (523.9908, -610.7643) centre (526.6325, -609.0031) ccw
  line L255 (523.9908, -610.7643) -> (565.6832, -673.303)
  arc A231 (526.5168, -637.4386) -> (520.7, -639.1998) centre (523.875, -639.1998) ccw
  line L256 (526.5168, -637.4386) -> (568.2092, -699.9773)
  line L257 (520.7, -701.7385) -> (520.7, -639.1998)
  arc A232 (520.7, -701.7385) -> (523.875, -704.9135) centre (523.875, -701.7385) ccw
  line L258 (565.5675, -704.9135) -> (523.875, -704.9135)
  arc A233 (565.5675, -704.9135) -> (568.2092, -699.9773) centre (565.5675, -701.7385) ccw
  line L259 (142.875, -717.6135) -> (184.5675, -717.6135)
  line L260 (187.2092, -722.5497) -> (145.5168, -785.0884)
  line L261 (139.7, -783.3272) -> (139.7, -720.7885)
  line L262 (142.9908, -811.7627) -> (184.6832, -749.224)
  line L263 (190.5, -750.9852) -> (190.5, -813.5239)
  line L264 (187.325, -816.6989) -> (145.6325, -816.6989)
  arc A234 (142.875, -717.6135) -> (139.7, -720.7885) centre (142.875, -720.7885) ccw
  arc A235 (187.2092, -722.5497) -> (184.5675, -717.6135) centre (184.5675, -720.7885) ccw
  arc A236 (139.7, -783.3272) -> (145.5168, -785.0884) centre (142.875, -783.3272) ccw
  arc A237 (190.5, -750.9852) -> (184.6832, -749.224) centre (187.325, -750.9852) ccw
  arc A238 (142.9908, -811.7627) -> (145.6325, -816.6989) centre (145.6325, -813.5239) ccw
  arc A239 (187.325, -816.6989) -> (190.5, -813.5239) centre (187.325, -813.5239) ccw
  line L265 (250.825, -717.6135) -> (209.1325, -717.6135)
  line L266 (206.4908, -722.5497) -> (248.1832, -785.0884)
  line L267 (254, -783.3272) -> (254, -720.7885)
  line L268 (250.7092, -811.7627) -> (209.0168, -749.224)
  line L269 (203.2, -750.9852) -> (203.2, -813.5239)
  line L270 (206.375, -816.6989) -> (248.0675, -816.6989)
  arc A240 (254, -720.7885) -> (250.825, -717.6135) centre (250.825, -720.7885) ccw
  arc A241 (209.1325, -717.6135) -> (206.4908, -722.5497) centre (209.1325, -720.7885) ccw
  arc A242 (248.1832, -785.0884) -> (254, -783.3272) centre (250.825, -783.3272) ccw
  arc A243 (209.0168, -749.224) -> (203.2, -750.9852) centre (206.375, -750.9852) ccw
  arc A244 (248.0675, -816.6989) -> (250.7092, -811.7627) centre (248.0675, -813.5239) ccw
  arc A245 (203.2, -813.5239) -> (206.375, -816.6989) centre (206.375, -813.5239) ccw
  line L271 (269.875, -717.6135) -> (311.5675, -717.6135)
  line L272 (314.2092, -722.5497) -> (272.5168, -785.0884)
  line L273 (266.7, -783.3272) -> (266.7, -720.7885)
  line L274 (269.9908, -811.7627) -> (311.6832, -749.224)
  line L275 (317.5, -750.9852) -> (317.5, -813.5239)
  line L276 (314.325, -816.6989) -> (272.6325, -816.6989)
  arc A246 (269.875, -717.6135) -> (266.7, -720.7885) centre (269.875, -720.7885) ccw
  arc A247 (314.2092, -722.5497) -> (311.5675, -717.6135) centre (311.5675, -720.7885) ccw
  arc A248 (266.7, -783.3272) -> (272.5168, -785.0884) centre (269.875, -783.3272) ccw
  arc A249 (317.5, -750.9852) -> (311.6832, -749.224) centre (314.325, -750.9852) ccw
  arc A250 (269.9908, -811.7627) -> (272.6325, -816.6989) centre (272.6325, -813.5239) ccw
  arc A251 (314.325, -816.6989) -> (317.5, -813.5239) centre (314.325, -813.5239) ccw
  arc A252 (336.1325, -717.6135) -> (333.4908, -722.5497) centre (336.1325, -720.7885) ccw
  line L277 (377.825, -717.6135) -> (336.1325, -717.6135)
  arc A253 (381, -720.7885) -> (377.825, -717.6135) centre (377.825, -720.7885) ccw
  line L278 (333.4908, -722.5497) -> (375.1832, -785.0884)
  arc A254 (336.0168, -749.224) -> (330.2, -750.9852) centre (333.375, -750.9852) ccw
  line L279 (381, -783.3272) -> (381, -720.7885)
  arc A255 (375.1832, -785.0884) -> (381, -783.3272) centre (377.825, -783.3272) ccw
  line L280 (377.7092, -811.7627) -> (336.0168, -749.224)
  arc A256 (375.0675, -816.6989) -> (377.7092, -811.7627) centre (375.0675, -813.5239) ccw
  line L281 (333.375, -816.6989) -> (375.0675, -816.6989)
  arc A257 (330.2, -813.5239) -> (333.375, -816.6989) centre (333.375, -813.5239) ccw
  line L282 (330.2, -750.9852) -> (330.2, -813.5239)
  line L283 (396.875, -717.6135) -> (438.5675, -717.6135)
  line L284 (441.2092, -722.5497) -> (399.5168, -785.0884)
  line L285 (393.7, -783.3272) -> (393.7, -720.7885)
  line L286 (396.9908, -811.7627) -> (438.6832, -749.224)
  line L287 (444.5, -750.9852) -> (444.5, -813.5239)
  line L288 (441.325, -816.6989) -> (399.6325, -816.6989)
  arc A258 (396.875, -717.6135) -> (393.7, -720.7885) centre (396.875, -720.7885) ccw
  arc A259 (441.2092, -722.5497) -> (438.5675, -717.6135) centre (438.5675, -720.7885) ccw
  arc A260 (393.7, -783.3272) -> (399.5168, -785.0884) centre (396.875, -783.3272) ccw
  arc A261 (444.5, -750.9852) -> (438.6832, -749.224) centre (441.325, -750.9852) ccw
  arc A262 (396.9908, -811.7627) -> (399.6325, -816.6989) centre (399.6325, -813.5239) ccw
  arc A263 (441.325, -816.6989) -> (444.5, -813.5239) centre (441.325, -813.5239) ccw
  arc A264 (463.1325, -717.6135) -> (460.4908, -722.5497) centre (463.1325, -720.7885) ccw
  line L289 (504.825, -717.6135) -> (463.1325, -717.6135)
  arc A265 (508, -720.7885) -> (504.825, -717.6135) centre (504.825, -720.7885) ccw
  line L290 (460.4908, -722.5497) -> (502.1832, -785.0884)
  arc A266 (463.0168, -749.224) -> (457.2, -750.9852) centre (460.375, -750.9852) ccw
  line L291 (508, -783.3272) -> (508, -720.7885)
  arc A267 (502.1832, -785.0884) -> (508, -783.3272) centre (504.825, -783.3272) ccw
  line L292 (504.7092, -811.7627) -> (463.0168, -749.224)
  arc A268 (502.0675, -816.6989) -> (504.7092, -811.7627) centre (502.0675, -813.5239) ccw
  line L293 (460.375, -816.6989) -> (502.0675, -816.6989)
  arc A269 (457.2, -813.5239) -> (460.375, -816.6989) centre (460.375, -813.5239) ccw
  line L294 (457.2, -750.9852) -> (457.2, -813.5239)
  arc A270 (523.875, -717.6135) -> (520.7, -720.7885) centre (523.875, -720.7885) ccw
  line L295 (523.875, -717.6135) -> (565.5675, -717.6135)
  arc A271 (568.2092, -722.5497) -> (565.5675, -717.6135) centre (565.5675, -720.7885) ccw
  line L296 (523.9908, -811.7627) -> (565.6832, -749.224)
  line L297 (571.5, -750.9852) -> (571.5, -813.5239)
  arc A272 (523.9908, -811.7627) -> (526.6325, -816.6989) centre (526.6325, -813.5239) ccw
  line L298 (568.325, -816.6989) -> (526.6325, -816.6989)
  arc A273 (568.325, -816.6989) -> (571.5, -813.5239) centre (568.325, -813.5239) ccw
  line L299 (520.7, -783.3272) -> (520.7, -720.7885)
  arc A274 (520.7, -783.3272) -> (526.5168, -785.0884) centre (523.875, -783.3272) ccw
  line L300 (568.2092, -722.5497) -> (526.5168, -785.0884)
  arc A275 (571.5, -750.9852) -> (565.6832, -749.224) centre (568.325, -750.9852) ccw
  point P0 (139.7, -46.9011)
  point P1 (139.7, -123.1011)
  point P2 (190.5, -46.9011)
  point P3 (190.5, -145.9865)
  point P4 (139.7, -145.9865)
  point P5 (190.5, -106.299)
  point P6 (254, -46.9011)
  point P7 (254, -123.1011)
  point P8 (203.2, -46.9011)
  point P9 (203.2, -69.7865)
  point P10 (203.2, -145.9865)
  point P11 (254, -145.9865)
  point P12 (203.2, -106.299)
  point P13 (139.7, -257.7719)
  point P14 (139.7, -181.5719)
  point P15 (190.5, -257.7719)
  point P16 (190.5, -158.6865)
  point P17 (139.7, -158.6865)
  point P18 (190.5, -198.374)
  point P19 (254, -257.7719)
  point P20 (203.2, -257.7719)
  point P21 (203.2, -234.8865)
  point P22 (203.2, -198.374)
  point P23 (254, -181.5719)
  point P24 (203.2, -158.6865)
  point P25 (254, -158.6865)
  point P26 (266.7, -46.9011)
  point P27 (266.7, -123.1011)
  point P28 (317.5, -46.9011)
  point P29 (317.5, -145.9865)
  point P30 (266.7, -145.9865)
  point P31 (317.5, -106.299)
  point P32 (381, -46.9011)
  point P33 (330.2, -46.9011)
  point P34 (330.2, -69.7865)
  point P35 (330.2, -106.299)
  point P36 (381, -123.1011)
  point P37 (330.2, -145.9865)
  point P38 (381, -145.9865)
  point P39 (317.5, -198.374)
  point P40 (317.5, -257.7719)
  point P41 (266.7, -257.7719)
  point P42 (330.2, -234.8865)
  point P43 (266.7, -181.5719)
  point P44 (317.5, -158.6865)
  point P45 (266.7, -158.6865)
  point P46 (330.2, -158.6865)
  point P47 (330.2, -198.374)
  point P48 (381, -181.5719)
  point P49 (381, -158.6865)
  point P50 (381, -257.7719)
  point P51 (330.2, -257.7719)
  point P52 (393.7, -46.9011)
  point P53 (393.7, -123.1011)
  point P54 (444.5, -46.9011)
  point P55 (444.5, -145.9865)
  point P56 (393.7, -145.9865)
  point P57 (444.5, -106.299)
  point P58 (508, -46.9011)
  point P59 (457.2, -46.9011)
  point P60 (457.2, -69.7865)
  point P61 (457.2, -106.299)
  point P62 (508, -123.1011)
  point P63 (457.2, -145.9865)
  point P64 (508, -145.9865)
  point P65 (444.5, -198.374)
  point P66 (444.5, -257.7719)
  point P67 (393.7, -257.7719)
  point P68 (457.2, -234.8865)
  point P69 (393.7, -181.5719)
  point P70 (444.5, -158.6865)
  point P71 (393.7, -158.6865)
  point P72 (457.2, -158.6865)
  point P73 (457.2, -198.374)
  point P74 (508, -181.5719)
  point P75 (508, -158.6865)
  point P76 (508, -257.7719)
  point P77 (457.2, -257.7719)
  point P78 (139.7, -270.4719)
  point P79 (139.7, -346.6719)
  point P80 (190.5, -270.4719)
  point P81 (190.5, -369.5573)
  point P82 (139.7, -369.5573)
  point P83 (190.5, -329.8698)
  point P84 (254, -270.4719)
  point P85 (203.2, -270.4719)
  point P86 (203.2, -293.3573)
  point P87 (203.2, -329.8698)
  point P88 (254, -346.6719)
  point P89 (203.2, -369.5573)
  point P90 (254, -369.5573)
  point P91 (190.5, -421.9448)
  point P92 (190.5, -481.3427)
  point P93 (139.7, -481.3427)
  point P94 (203.2, -458.4573)
  point P95 (139.7, -405.1427)
  point P96 (190.5, -382.2573)
  point P97 (139.7, -382.2573)
  point P98 (203.2, -382.2573)
  point P99 (203.2, -421.9448)
  point P100 (254, -405.1427)
  point P101 (254, -382.2573)
  point P102 (254, -481.3427)
  point P103 (203.2, -481.3427)
  point P104 (266.7, -270.4719)
  point P105 (266.7, -346.6719)
  point P106 (317.5, -270.4719)
  point P107 (317.5, -369.5573)
  point P108 (266.7, -369.5573)
  point P109 (317.5, -329.8698)
  point P110 (381, -270.4719)
  point P111 (330.2, -270.4719)
  point P112 (330.2, -293.3573)
  point P113 (330.2, -329.8698)
  point P114 (381, -346.6719)
  point P115 (330.2, -369.5573)
  point P116 (381, -369.5573)
  point P117 (317.5, -421.9448)
  point P118 (317.5, -481.3427)
  point P119 (266.7, -481.3427)
  point P120 (330.2, -458.4573)
  point P121 (266.7, -405.1427)
  point P122 (317.5, -382.2573)
  point P123 (266.7, -382.2573)
  point P124 (330.2, -382.2573)
  point P125 (330.2, -421.9448)
  point P126 (381, -405.1427)
  point P127 (381, -382.2573)
  point P128 (381, -481.3427)
  point P129 (330.2, -481.3427)
  point P130 (393.7, -270.4719)
  point P131 (393.7, -346.6719)
  point P132 (444.5, -270.4719)
  point P133 (444.5, -369.5573)
  point P134 (393.7, -369.5573)
  point P135 (444.5, -329.8698)
  point P136 (508, -270.4719)
  point P137 (457.2, -270.4719)
  point P138 (457.2, -293.3573)
  point P139 (457.2, -329.8698)
  point P140 (508, -346.6719)
  point P141 (457.2, -369.5573)
  point P142 (508, -369.5573)
  point P143 (444.5, -421.9448)
  point P144 (444.5, -481.3427)
  point P145 (393.7, -481.3427)
  point P146 (457.2, -458.4573)
  point P147 (393.7, -405.1427)
  point P148 (444.5, -382.2573)
  point P149 (393.7, -382.2573)
  point P150 (457.2, -382.2573)
  point P151 (457.2, -421.9448)
  point P152 (508, -405.1427)
  point P153 (508, -382.2573)
  point P154 (508, -481.3427)
  point P155 (457.2, -481.3427)
  point P156 (139.7, -494.0427)
  point P157 (139.7, -570.2427)
  point P158 (190.5, -494.0427)
  point P159 (190.5, -593.1281)
  point P160 (139.7, -593.1281)
  point P161 (190.5, -553.4406)
  point P162 (254, -494.0427)
  point P163 (203.2, -494.0427)
  point P164 (203.2, -516.9281)
  point P165 (203.2, -553.4406)
  point P166 (254, -570.2427)
  point P167 (203.2, -593.1281)
  point P168 (254, -593.1281)
  point P169 (190.5, -645.5156)
  point P170 (190.5, -704.9135)
  point P171 (139.7, -704.9135)
  point P172 (203.2, -682.0281)
  point P173 (139.7, -628.7135)
  point P174 (190.5, -605.8281)
  point P175 (139.7, -605.8281)
  point P176 (203.2, -605.8281)
  point P177 (203.2, -645.5156)
  point P178 (254, -628.7135)
  point P179 (254, -605.8281)
  point P180 (254, -704.9135)
  point P181 (203.2, -704.9135)
  point P182 (266.7, -494.0427)
  point P183 (266.7, -570.2427)
  point P184 (317.5, -494.0427)
  point P185 (317.5, -593.1281)
  point P186 (266.7, -593.1281)
  point P187 (317.5, -553.4406)
  point P188 (381, -494.0427)
  point P189 (330.2, -494.0427)
  point P190 (330.2, -516.9281)
  point P191 (330.2, -553.4406)
  point P192 (381, -570.2427)
  point P193 (330.2, -593.1281)
  point P194 (381, -593.1281)
  point P195 (317.5, -645.5156)
  point P196 (317.5, -704.9135)
  point P197 (266.7, -704.9135)
  point P198 (330.2, -682.0281)
  point P199 (266.7, -628.7135)
  dimension "d0" = 711.2
  dimension "d1" = 863.6
  dimension "d2" = 50.8
  dimension "d3" = 76.2
  dimension "d4" = 50.8
  dimension "d5" = 76.2
  dimension "d6" = 22.8854
  dimension "d7" = 139.7
  dimension "d8" = 46.9011
  dimension "d9" = 6.35
  dimension "d10" = 3.175
  dimension "d11" = 6.35
  dimension "d14" = 127
  dimension "d17" = 223.5708
  dimension "d20" = 6.35
  dimension "d22" = 76.2
  dimension "d23" = 50.8
  dimension "d24" = 22.8854
  dimension "d25" = 50.8
  dimension "d26" = 12.7
  dimension "d27" = 3.175
  dimension "d30" = 127
  constraints: 602 end point, 552 point on circle, 538 point on line, 276 centre point, 254 symmetric about line, 34 tangent, 15 equal radius, 6 horizontal, 5 parallel, 4 midpoint, 4 perpendicular, 4 vertical, 3 vertical alignment, 1 coincident, 1327 other
  measures "d0" distance of L0.start L0.end
  measures "d1" distance of L2.end L0.start
  measures "d2" distance of point (190.5, -46.901) point (139.7, -46.901)
  measures "d3" distance of point (139.7, -46.901) point (139.7, -123.101)
  measures "d4" distance of point (190.5, -145.986) point (139.7, -145.986)
  measures "d5" distance of L7.start point (190.5, -145.986)
  measures "d6" distance of point (139.7, -145.986) point (139.7, -123.101)
  measures "d7" distance between parallel lines of L3 L4
  measures "d8" distance between parallel lines of L0 L6
  measures "d9" distance between parallel lines of L7 L10
  measures "d10" radius of A0
  measures "d11" distance between parallel lines of L15 L17
  measures "d14" distance of L21.start L43.end
  measures "d17" distance of L21.start L91.end
  measures "d20" distance between parallel lines of L222 L205
  measures "d22" distance of point (139.7, -793.814) point (139.7, -717.614)
  measures "d23" distance of point (139.7, -717.614) point (190.5, -717.614)
  measures "d24" distance of point (139.7, -793.814) point (139.7, -816.699)
  measures "d25" distance of point (190.5, -816.699) point (139.7, -816.699)
  measures "d26" distance between parallel lines of L165 L259
  measures "d27" radius of A234
  measures "d30" distance of point (203.2, -717.614) point (330.2, -717.614)
extrude "Extrusion1" add sketch "Sketch1" along normal blind 2.286